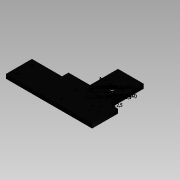
# Autodesk Inventor part: DudukanExt
Saved by Autodesk Inventor 2015 SP1 (Build 190203100, 203)
## iProperties
Created: 2015-02-03
Part Number: DudukanExt
Material: Generic
Document SubType Name: Modeling
Designer: Rafi Kurnia Putra
Density: 1 g/cm^3
Appearance: Smooth - Purple
Mass: 19.4617 g
Surface Area: 130.296 cm^2
Volume: 19.4617 cm^3
Author: Rafi Kurnia Putra
Autodesk Inventor part; units mm, degrees
ref_plane "XZ Plane" through (0, 0, 0) normal (0, 1, 0) x (-1, 0, 0)
sketch "Sketch1" plane through (0, 0, 0) normal (0, 1, 0) x (-1, 0, 0)
  line L0 (43.1973, 3.7398) -> (-56.8027, 3.7398)
  line L1 (-56.8027, 3.7398) -> (-56.8027, -26.2602)
  line L2 (43.1973, 3.7398) -> (43.1973, -26.2602)
  line L3 (-21.8027, -26.2602) -> (8.1973, -26.2602)
  line L4 (43.1973, -26.2602) -> (8.1973, -26.2602)
  line L5 (-21.8027, -26.2602) -> (-56.8027, -26.2602)
  line L6 (-21.8027, 3.7398) -> (8.1973, 3.7398)
  point P0 (0, 0)
  dimension "d2" = 100
  dimension "d6" = 30
  constraints: 14 end point, 3 horizontal, 3 perpendicular, 1 point on line, 1 vertical
  measures "d2" distance of L0.start L0.end
  measures "d6" distance of L0.end L1.end
extrude "Extrusion1" add sketch "Sketch1" along normal blind 5
sketch "Sketch4" plane through (0, 5, 0) normal (0, 1, 0) x (1, 0, 0)
  circle A0 centre (-36.6973, 2.7602) radius 1.75 projected
  circle A1 centre (-36.6973, 19.7602) radius 1.75 projected
  circle A2 centre (14.0028, 2.7602) radius 1.75 projected
  circle A3 centre (14.0028, 19.7602) radius 1.75 projected
  point P0 (0, 0)
extrude "Extrusion3" cut sketch "Sketch4" against normal through all
sketch "Sketch5" plane through (0, 0, 0) normal (0, -1, 0) x (1, 0, 0)
  circle A0 centre (41.8754, -14.1565) radius 1.5
  circle A1 centre (48.1213, -10.8415) radius 1.5
  circle A2 centre (44.8063, -4.5956) radius 1.5
  circle A3 centre (38.5604, -7.9106) radius 1.5
  line L0 (44.8063, -4.5956) -> (48.1213, -10.8415) construction
  line L1 (48.1213, -10.8415) -> (41.8754, -14.1565) construction
  line L2 (41.8754, -14.1565) -> (38.5604, -7.9106) construction
  line L3 (38.5604, -7.9106) -> (44.8063, -4.5956) construction
  line L4 (44.8063, -4.5956) -> (41.8754, -14.1565) construction
  line L5 (48.1213, -10.8415) -> (38.5604, -7.9106) construction
  line L6 (43.3409, -9.376) -> (52.1686, -4.6925)
  point P0 (0, 0)
  dimension "d47" = 3
  dimension "d48" = 3
  dimension "d49" = 3
  dimension "d50" = 3
  dimension "d51" = 3.315
  dimension "d52" = 3.315
  dimension "d53" = 7.0711
  dimension "d54" = 7.0711
  dimension "d55" = 7.0711
  dimension "d56" = 7.0711
  constraints: 14 end point, 4 centre point, 3 perpendicular, 1 midpoint
  measures "d47" diameter of A1
  measures "d48" diameter of A0
  measures "d49" diameter of A3
  measures "d50" diameter of A2
  measures "d51" horizontal distance of L0.start L0.end
  measures "d52" horizontal distance of L1.end L2.end
  measures "d53" distance of L0.start L0.end
  measures "d54" distance of L1.end L2.end
  measures "d55" distance of L2.end L0.start
  measures "d56" distance of L0.end L1.end
extrude "Extrusion4" cut sketch "Sketch5" against normal up to next
sketch "Sketch6" plane through (0, 0, 0) normal (0, -1, 0) x (1, 0, 0)
  circle A0 centre (6.7527, 80.0276) radius 4.235 projected
  circle A1 centre (6.7527, 80.0276) radius 4.8512
  point P0 (0, 0)
  dimension "d19" = 0.6162
  constraints: 1 centre point
  measures "d19" radial gap between concentric circles of A0 A1
sketch "Sketch7" plane through (-43.1973, 0, 3.7398) normal (0, 0, 1) x (1, 0, 0)
  line L0 (0, 0) -> (100, 0) projected
  line L1 (100, 0) -> (100, 5) projected
  line L2 (0, 5) -> (100, 5) projected
  line L3 (0, 0) -> (0, 5) projected
  line L4 (65, 0) -> (35, 0)
  line L5 (35, 0) -> (35, 5)
  line L6 (35, 5) -> (65, 5)
  line L7 (65, 5) -> (65, 0)
  line L8 (65, 0) -> (35, 5) construction
  line L9 (35, 0) -> (65, 5) construction
  point P0 (43.1973, 0)
  point P1 (50, 2.5)
  dimension "d22" = 30
  dimension "d23" = 5
  dimension "d24" = 6.8027
  dimension "d57" = 0
  constraints: 12 end point, 2 midpoint, 2 parallel, 1 horizontal, 1 perpendicular
  measures "d22" distance of L5.end L6.end
  measures "d23" distance of L4.end L5.end
  measures "d24" horizontal distance of point (50, 2.5) point (43.197, 0)
  measures "d57" distance between parallel lines of L4 L0
ref_plane "Work Plane2" through (6.8027, 0, 0) normal (1, 0, 0) x (0, 1, 0)
sketch "Sketch9" plane through (6.8027, 0, 0) normal (1, 0, 0) x (0, 1, 0)
  line L0 (2.5, 3.7398) -> (2.5, 8.7398)
  line L1 (2.5, 3.7398) -> (7.5, 3.7398) construction
  line L2 (2.5, 8.7398) -> (27.5, 8.7398)
  line L3 (27.5, 8.7398) -> (27.5, 88.7398)
  point P0 (0, 0)
  dimension "d26" = 5
  dimension "d27" = 90
  dimension "d28" = 25
  dimension "d29" = 80
  constraints: 8 end point, 3 perpendicular, 1 horizontal, 1 vertical
  measures "d26" distance of L0.start L0.end
  measures "d27" angle of L1 L0
  measures "d28" distance of L0.end L2.end
  measures "d29" distance of L2.end L3.end
sweep "Sweep1" add profiles "Sketch7" path "Sketch9" contours L5 L2 L7 L0
ref_plane "YZ 0" through (6.803, 0, 0) normal (1, 0, 0) x (0, 1, 0)
ref_plane "XY 0" through (0, 0, -11.25) normal (0, 0, 1) x (1, 0, 0)
sketch "Sketch12" plane through (-8.1973, 25, 11.2398) normal (0, -1, 0) x (1, 0, 0)
  circle A0 centre (15.0003, 42.485) radius 1.11
  point P0 (8.1973, -11.2398)
  constraints: 1 centre point, 2 other
extrude "Extrusion8" cut sketch "Sketch12" against normal up to next
sketch "Sketch13" plane through (-8.1973, 30, 6.2398) normal (0, 1, 0) x (1, 0, 0)
  circle A0 centre (15.0003, -45.985) radius 1.4
  point P0 (8.1973, 6.2398)
  constraints: 1 centre point, 2 other
extrude "Extrusion9" cut sketch "Sketch13" against normal up to next
sketch "Sketch15" plane through (-8.1973, 30, 6.2398) normal (0, 1, 0) x (1, 0, 0)
  circle A0 centre (15, -40) radius 4.5
  point P0 (8.1973, 6.2398)
  dimension "d40" = 9
  constraints: 1 centre point
  measures "d40" diameter of A0
extrude "Extrusion10" cut sketch "Sketch15" against normal up to next
sketch "Sketch16" plane through (-8.1973, 25, 11.2398) normal (0, -1, 0) x (1, 0, 0)
  circle A0 centre (15, 42.5) radius 12
  line L0 (30, 0) -> (30, 77.5) projected
  line L1 (0, 0) -> (0, 77.5) projected
  line L2 (30, 77.5) -> (0, 77.5)
  line L3 (0, 77.5) -> (0, 57.5)
  line L4 (0, 57.5) -> (30, 57.5)
  line L5 (30, 57.5) -> (30, 77.5)
  point P0 (8.1973, -11.2398)
  point P1 (15, 57.5)
  dimension "d43" = 15
  dimension "d44" = 15
  constraints: 8 end point, 2 parallel, 1 centre point, 1 horizontal, 1 perpendicular, 1 point on line, 2 other
  measures "d43" distance from line of A0.centre L0
  measures "d44" distance of point (15, 57.5) A0.centre
extrude "Extrusion11" cut sketch "Sketch16" against normal up to next contours L4 L1 L2 L0
sketch "Sketch17" plane through (-8.1973, 30, 6.2398) normal (0, 1, 0) x (1, 0, 0)
  circle A0 centre (8.9896, -46.0153) radius 1.25
  circle A1 centre (8.9896, -33.9945) radius 1.25
  circle A2 centre (21.0104, -46.0153) radius 1.25
  circle A3 centre (21.0104, -33.9945) radius 1.25
  line L0 (8.9896, -46.0153) -> (8.9896, -33.9945) construction
  line L1 (8.9896, -33.9945) -> (21.0104, -33.9945) construction
  line L2 (21.0104, -33.9945) -> (21.0104, -46.0153) construction
  line L3 (21.0104, -46.0153) -> (8.9896, -46.0153) construction
  line L4 (21.0104, -33.9945) -> (8.9896, -46.0153) construction
  line L5 (8.9896, -33.9945) -> (21.0104, -46.0153) construction
  line L6 (0, -62.5) -> (30, -62.5) construction
  line L7 (0, 0) -> (0, -62.5) construction
  line L8 (30, 0) -> (30, -62.5) construction
  point P0 (8.1973, 6.2398)
  dimension "d64" = 12.0208
  dimension "d65" = 12.0208
  dimension "d66" = 12.0208
  dimension "d67" = 12.0208
  dimension "d68" = 17
  dimension "d69" = 17
  dimension "d70" = 2.5
  dimension "d71" = 2.5
  dimension "d72" = 2.5
  dimension "d73" = 2.5
  constraints: 12 end point, 4 centre point, 4 perpendicular, 3 parallel, 1 vertical
  measures "d64" distance of L0.end L0.start
  measures "d65" distance of L1.end L2.end
  measures "d66" distance of L1.end L0.end
  measures "d67" distance of L2.end L0.start
  measures "d68" distance of L1.end L0.start
  measures "d69" distance of L2.end L0.end
  measures "d70" diameter of A1
  measures "d71" diameter of A0
  measures "d72" diameter of A2
  measures "d73" diameter of A3
extrude "Extrusion12" cut sketch "Sketch17" against normal up to next
sketch "Sketch18" plane through (6.803, 0, 0) normal (1, 0, 0) x (0, 1, 0)
  line L0 (25, 11.2398) -> (15, 11.2398)
  line L1 (0, 11.2398) -> (25, 11.2398) projected
  line L2 (25, 11.2398) -> (25, 21.2398)
  line L3 (25, 11.2398) -> (25, 68.7398) projected
  line L4 (25, 21.2398) -> (15, 11.2398)
  point P0 (0, 0)
  dimension "d76" = 10
  dimension "d79" = 10
  constraints: 6 end point, 2 point on line
  measures "d76" distance of L0.start L2.end
  measures "d79" distance of L0.start L0.end
extrude "Extrusion13" add sketch "Sketch18" along normal mid plane 30
sketch "Sketch19" plane through (6.803, 0, 0) normal (1, 0, 0) x (0, 1, 0)
  line L0 (5, 6.2398) -> (7.5, 6.2398)
  line L1 (5, 6.2398) -> (30, 6.2398) projected
  line L2 (5, 6.2398) -> (7.5, 6.2398) construction
  line L3 (7.5, 6.2398) -> (5, 3.7398)
  line L4 (5, 3.7398) -> (5, 6.2398)
  point P0 (0, 0)
  dimension "d80" = 2.5
  dimension "d81" = 0
  dimension "d82" = 45
  constraints: 8 end point, 2 collinear, 1 horizontal, 1 perpendicular
  measures "d80" distance of L0.start L0.end
  measures "d81" distance between parallel lines of L0 L2
  measures "d82" angle of L0 L3
extrude "Extrusion14" add sketch "Sketch19" along normal mid plane 30
sketch "Sketch20" plane through (-8.1973, 30, 6.2398) normal (0, 1, 0) x (1, 0, 0)
  circle A0 centre (15, -40) radius 4.5 projected
  arc A1 (15.9875, -46.9776) -> (14.013, -46.9776) centre (15.0003, -45.985) ccw projected
  arc A2 (14.013, -46.9776) -> (15.9875, -46.9776) centre (15.0003, -47.485) ccw projected
  point P0 (8.1973, 6.2398)
extrude "Extrusion15" add sketch "Sketch20" against normal blind 5 contours A2 A1
equation "\"d71\" = d70"
equation "\"d72\" = d70"
equation "\"d73\" = d70"
body "Solid1"
